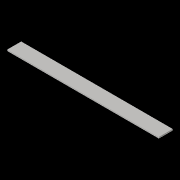
# Autodesk Inventor part: NMMCMARK2
Saved by Autodesk Inventor 2016 (Build 200138000, 138)
## iProperties
Created: 2017-01-28
Part Number: NMMCMARK2
Material: Generic
Document SubType Name: Modeling
Designer: Alexis Renderos
Density: 1 g/cm^3
Appearance: Default
Author: Alexis Renderos
Autodesk Inventor part; units mm, degrees
ref_plane "YZ Plane" through (0, 0, 0) normal (1, 0, 0) x (0, 1, 0)
ref_plane "XZ Plane" through (0, 0, 0) normal (0, 1, 0) x (-1, 0, 0)
ref_plane "XY Plane" through (0, 0, 0) normal (0, 0, 1) x (1, 0, 0)
sketch "Sketch1" plane through (0, 0, 0) normal (0, 1, 0) x (-1, 0, 0)
  line L0 (0, -44.45) -> (0, 44.45) projected
  line L1 (-493.715, 0) -> (493.715, 0) projected
  line L2 (352.6536, -31.75) -> (-352.6536, -31.75)
  line L3 (-352.6536, -31.75) -> (-352.6536, 31.75)
  line L4 (-352.6536, 31.75) -> (352.6536, 31.75)
  line L5 (352.6536, 31.75) -> (352.6536, -31.75)
  point P0 (0, 0)
  dimension "d0" = 705.3072
  dimension "d1" = 63.5
  constraints: 8 end point, 2 parallel, 1 horizontal, 1 perpendicular, 2 other
  measures "d0" distance of L4.end L3.end
  measures "d1" distance of L3.end L2.end
extrude "Extrusion1" add sketch "Sketch1" along normal mid plane 6.35
body "Solid1"
